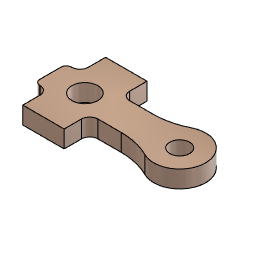
12lb power swich (Autodesk Fusion 360 archive; units mm, degrees)
design "copper thing_large hole"
Autodesk Fusion 360 part; units mm, degrees
sketch "Sketch1" plane through (0, 0, 0) normal (0, 1, 0) x (1, 0, 0)
  circle A0 centre (0, 0) radius 2.3876
  line L0 (-6.35, -2.921) -> (22.225, -2.921)
  line L1 (22.225, -2.921) -> (22.225, 2.921)
  line L2 (22.225, 2.921) -> (-6.35, 2.921)
  line L3 (-6.35, 2.921) -> (-6.35, -2.921)
  line L4 (-6.35, 0) -> (22.225, 0) construction
  circle A1 centre (17.4498, 0) radius 1.8288
  line L5 (9.525, 2.921) -> (9.525, -2.921) construction
  circle A2 centre (17.4498, 0) radius 4.7752
  line L6 (3.81, -7.62) -> (-3.81, -7.62)
  line L7 (-3.81, -7.62) -> (-3.81, 7.62)
  line L8 (-3.81, 7.62) -> (3.81, 7.62)
  line L9 (3.81, 7.62) -> (3.81, -7.62)
  line L10 (3.81, -7.62) -> (-3.81, 7.62) construction
  line L11 (-3.81, -7.62) -> (3.81, 7.62) construction
  dimension "d1" = 4.7752
  dimension "d2" = 28.575
  dimension "d3" = 5.842
  dimension "d5" = 6.35
  dimension "d6" = 3.6576
  dimension "d7" = 4.7752
  dimension "d8" = 9.525
  dimension "d24" = 7.62
  dimension "d25" = 15.24
  constraint coincident A0.centre origin
  constraint horizontal L0
  constraint vertical L1
  constraint horizontal L2
  constraint vertical L3
  constraint midpoint L3 L4.start
  constraint midpoint L1 L4.end
  constraint coincident A0.centre L4
  constraint coincident L4 A1.centre
  constraint coincident L2 L5.start
  constraint coincident L0 L5.end
  constraint perpendicular L0 L5
  constraint concentric A1 A2
  constraint coincident L4.end A2
  constraint horizontal L6
  constraint perpendicular L6 L7
  constraint parallel L6 L8
  constraint parallel L7 L9
  constraint coincident L10 A0.centre
  constraint coincident L11 A0.centre
  measures "d1" diameter of A0
  measures "d2" distance of L0.start L0.end
  measures "d3" distance of L0.end L1.end
  measures "d5" distance of A0.centre L3
  measures "d6" diameter of A1
  measures "d7" distance of L4.end A1.centre
  measures "d8" distance of A0.centre L5
  measures "d24" distance of L7.end L8.end
  measures "d25" distance of L6.end L7.end
extrude "Extrude1" add sketch "Sketch1" along normal blind 3.175 contours L0 L2 L3 L7 | L0 L2 L7 L9 | L0 L6 L7 L9 | L0 L2 A2 L9 | L2 L7 L8 L9 | L0 L2 A2 | L0 A2 | L2 A2
fillet "Fillet2" radius 0.9652 2 edges at (-6.35, 1.5875, 2.921) (-6.35, 1.5875, -2.921)
fillet "Fillet4" radius 12.7 2 edges at (13.6722, 1.5875, 2.921) (13.6722, 1.5875, -2.921)
fillet "Fillet6" radius 1.5 4 edges at (-3.81, 1.5875, 2.921) (3.81, 1.5875, 2.921) (3.81, 1.5875, -2.921) (-3.81, 1.5875, -2.921)
equation "d3 = ( 0.115 * 2 ) * 1 in"

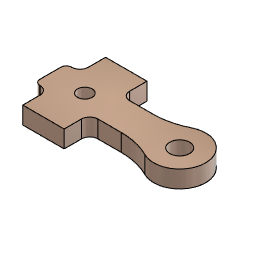
design "copper thing_Tapped"
Autodesk Fusion 360 part; units mm, degrees
sketch "Sketch1" plane through (0, 0, 0) normal (0, 1, 0) x (1, 0, 0)
  circle A0 centre (0, 0) radius 1.3525
  line L0 (-6.35, -2.921) -> (22.225, -2.921)
  line L1 (22.225, -2.921) -> (22.225, 2.921)
  line L2 (22.225, 2.921) -> (-6.35, 2.921)
  line L3 (-6.35, 2.921) -> (-6.35, -2.921)
  line L4 (-6.35, 0) -> (22.225, 0) construction
  circle A1 centre (17.4498, 0) radius 1.8288
  line L5 (9.525, 2.921) -> (9.525, -2.921) construction
  circle A2 centre (17.4498, 0) radius 4.7752
  line L6 (3.81, -7.62) -> (-3.81, -7.62)
  line L7 (-3.81, -7.62) -> (-3.81, 7.62)
  line L8 (-3.81, 7.62) -> (3.81, 7.62)
  line L9 (3.81, 7.62) -> (3.81, -7.62)
  line L10 (3.81, -7.62) -> (-3.81, 7.62) construction
  line L11 (-3.81, -7.62) -> (3.81, 7.62) construction
  dimension "d1" = 2.7051
  dimension "d2" = 28.575
  dimension "d3" = 5.842
  dimension "d5" = 6.35
  dimension "d6" = 3.6576
  dimension "d7" = 4.7752
  dimension "d8" = 9.525
  dimension "d24" = 7.62
  dimension "d25" = 15.24
  constraint coincident A0.centre origin
  constraint horizontal L0
  constraint vertical L1
  constraint horizontal L2
  constraint vertical L3
  constraint midpoint L3 L4.start
  constraint midpoint L1 L4.end
  constraint coincident A0.centre L4
  constraint coincident L4 A1.centre
  constraint coincident L2 L5.start
  constraint coincident L0 L5.end
  constraint perpendicular L0 L5
  constraint concentric A1 A2
  constraint coincident L4.end A2
  constraint horizontal L6
  constraint perpendicular L6 L7
  constraint parallel L6 L8
  constraint parallel L7 L9
  constraint coincident L10 A0.centre
  constraint coincident L11 A0.centre
  measures "d1" diameter of A0
  measures "d2" distance of L0.start L0.end
  measures "d3" distance of L0.end L1.end
  measures "d5" distance of A0.centre L3
  measures "d6" diameter of A1
  measures "d7" distance of L4.end A1.centre
  measures "d8" distance of A0.centre L5
  measures "d24" distance of L7.end L8.end
  measures "d25" distance of L6.end L7.end
extrude "Extrude1" add sketch "Sketch1" along normal blind 3.175 contours L0 L2 L3 L7 | L0 L2 L7 L9 | L0 L6 L7 L9 | L0 L2 A2 L9 | L2 L7 L8 L9 | L0 L2 A2 | L0 A2 | L2 A2
fillet "Fillet2" radius 0.9652 2 edges at (-6.35, 1.5875, 2.921) (-6.35, 1.5875, -2.921)
fillet "Fillet4" radius 12.7 2 edges at (13.6722, 1.5875, 2.921) (13.6722, 1.5875, -2.921)
fillet "Fillet6" radius 1.5 4 edges at (3.81, 1.5875, 2.921) (3.81, 1.5875, -2.921) (-3.81, 1.5875, -2.921) (-3.81, 1.5875, 2.921)
equation "d3 = ( 0.115 * 2 ) * 1 in"
